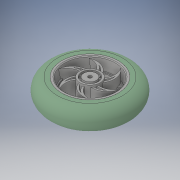
# Autodesk Inventor part: Wheel Hub
Saved by Autodesk Inventor 2018 (Build 220112000, 112)
## iProperties
Created: 2018-03-28
Part Number: Wheel Hub
Material: Generic
Document SubType Name: Modeling
Designer: Ajith Thomas
Density: 1 g/cm^3
Appearance: Default
Author: Ajith Thomas
Autodesk Inventor part; units mm, degrees
ref_plane "YZ Plane" through (0, 0, 0) normal (1, 0, 0) x (0, 1, 0)
sketch "Sketch1" plane through (0, 0, 0) normal (0, 1, 0) x (-1, 0, 0)
  circle A0 centre (0, 0) radius 23.5
  dimension "d0" = 47
  constraints: 1 centre point, 1 coincident
  measures "d0" diameter of A0
extrude "Extrusion1" add sketch "Sketch1" along normal blind 19
sketch "Sketch2" plane through (0, 19, 0) normal (0, 1, 0) x (1, 0, 0)
  circle A0 centre (0, 0) radius 21.25
  dimension "d3" = 42.5
  constraints: 1 centre point, 1 coincident
  measures "d3" diameter of A0
extrude "Extrusion2" cut sketch "Sketch2" against normal blind 19
sketch "Sketch3" plane through (0, 19, 0) normal (0, 1, 0) x (1, 0, 0)
  circle A0 centre (0, 0) radius 5.25
  dimension "d6" = 10.5
  constraints: 1 centre point, 1 coincident
  measures "d6" diameter of A0
extrude "Extrusion3" add sketch "Sketch3" against normal blind 19
sketch "Sketch4" plane through (0, 19, 0) normal (0, 1, 0) x (1, 0, 0)
  circle A0 centre (0, 0) radius 1.5
  dimension "d9" = 3
  constraints: 1 centre point, 1 coincident
  measures "d9" diameter of A0
extrude "Extrusion4" cut sketch "Sketch4" against normal blind 19
ref_plane "Work Plane1" through (0, 9.5, 0) normal (0, 1, 0) x (1, 0, 0)
sketch "Sketch5" plane through (0, 9.5, 0) normal (0, 1, 0) x (1, 0, 0)
  circle A0 centre (0, 0) radius 5.25 projected
  circle A1 centre (0, 0) radius 21.25 projected
  line L0 (-21.25, 0) -> (0, 0) construction
  line L1 (0, 0) -> (21.25, 0) construction
  circle A2 centre (0, 0) radius 1.5 construction
  line L2 (0, -21.25) -> (0, 0) construction
  line L3 (0, 0) -> (0, 21.25) construction
  arc A3 (-2.2887, 4.7249) -> (-15.5928, 14.437) centre (-13.6129, 3.1808) ccw
  arc A4 (2.8284, 4.4229) -> (-15.5928, 14.437) centre (-10.0016, 2.772) ccw
  arc A5 (2.8284, 4.4229) -> (-2.2887, 4.7249) centre (0, 0) ccw
  arc A6 (-2.4162, 4.661) -> (-5.2362, 0.3804) centre (0, 0) ccw
  arc A7 (-5.2362, 0.3804) -> (-20.2992, -6.2853) centre (-9.5611, -10.1987) ccw
  arc A8 (-2.4162, 4.661) -> (-20.2992, -6.2853) centre (-7.4014, -7.2756) ccw
  arc A9 (-5.2446, 0.238) -> (-2.9475, -4.3445) centre (0, 0) ccw
  arc A10 (-2.9475, -4.3445) -> (-4.7064, -20.7223) centre (4.0518, -13.3795) ccw
  arc A11 (-5.2446, 0.238) -> (-4.7064, -20.7223) centre (2.6002, -10.0476) ccw
  arc A12 (-2.8284, -4.4229) -> (2.2887, -4.7249) centre (0, 0) ccw
  arc A13 (2.2887, -4.7249) -> (15.5928, -14.437) centre (13.6129, -3.1808) ccw
  arc A14 (-2.8284, -4.4229) -> (15.5928, -14.437) centre (10.0016, -2.772) ccw
  arc A15 (2.4162, -4.661) -> (5.2362, -0.3804) centre (0, 0) ccw
  arc A16 (5.2362, -0.3804) -> (20.2992, 6.2853) centre (9.5611, 10.1987) ccw
  arc A17 (2.4162, -4.661) -> (20.2992, 6.2853) centre (7.4014, 7.2756) ccw
  arc A18 (5.2446, -0.238) -> (2.9475, 4.3445) centre (0, 0) ccw
  arc A19 (2.9475, 4.3445) -> (4.7064, 20.7223) centre (-4.0518, 13.3795) ccw
  arc A20 (5.2446, -0.238) -> (4.7064, 20.7223) centre (-2.6002, 10.0476) ccw
  dimension "d14" = 360
  constraints: 43 point on circle, 18 centre point, 8 end point, 2 point on line, 1 horizontal, 1 vertical, 55 other
extrude "Extrusion5" add sketch "Sketch5" along normal mid plane 16 contours A0 A19 A20 | A0 A3 A4 | A16 A17 A0 | A0 A7 A8 | A13 A14 A0 | A11 A0 A10
sketch "Sketch6" plane through (0, 17.5, 0) normal (0, 1, 0) x (1, 0, 0)
  arc A0 (-2.2887, 4.7249) -> (-15.5928, 14.437) centre (-13.6129, 3.1808) ccw projected
  arc A1 (2.8284, 4.4229) -> (-15.5928, 14.437) centre (-10.0016, 2.772) ccw projected
  arc A2 (2.8284, 4.4229) -> (-2.2887, 4.7249) centre (0, 0) ccw projected
  arc A3 (2.8284, 4.4229) -> (-15.5928, 14.437) centre (-10.0016, 2.772) ccw projected
  arc A4 (-2.2887, 4.7249) -> (-15.5928, 14.437) centre (-13.6129, 3.1808) ccw projected
  arc A5 (-0.9458, 5.1641) -> (-6.2823, 13.6998) centre (-13.6129, 3.1808) ccw
  arc A6 (1.3079, 5.0845) -> (-6.2823, 13.6998) centre (-10.0016, 2.772) ccw
  arc A7 (1.3079, 5.0845) -> (-0.9458, 5.1641) centre (0, 0) ccw
  arc A8 (-3.7494, 3.6749) -> (-4.9452, 1.7629) centre (0, 0) ccw
  arc A9 (-4.9452, 1.7629) -> (-15.0055, 1.4093) centre (-9.5611, -10.1987) ccw
  arc A10 (-3.7494, 3.6749) -> (-15.0055, 1.4093) centre (-7.4014, -7.2756) ccw
  arc A11 (-5.0572, -1.4096) -> (-3.9993, -3.4012) centre (0, 0) ccw
  arc A12 (-3.9993, -3.4012) -> (-8.7232, -12.2905) centre (4.0518, -13.3795) ccw
  arc A13 (-5.0572, -1.4096) -> (-8.7232, -12.2905) centre (2.6002, -10.0476) ccw
  arc A14 (-1.3079, -5.0845) -> (0.9458, -5.1641) centre (0, 0) ccw
  arc A15 (0.9458, -5.1641) -> (6.2823, -13.6998) centre (13.6129, -3.1808) ccw
  arc A16 (-1.3079, -5.0845) -> (6.2823, -13.6998) centre (10.0016, -2.772) ccw
  arc A17 (3.7494, -3.6749) -> (4.9452, -1.7629) centre (0, 0) ccw
  arc A18 (4.9452, -1.7629) -> (15.0055, -1.4093) centre (9.5611, 10.1987) ccw
  arc A19 (3.7494, -3.6749) -> (15.0055, -1.4093) centre (7.4014, 7.2756) ccw
  arc A20 (5.0572, 1.4096) -> (3.9993, 3.4012) centre (0, 0) ccw
  arc A21 (3.9993, 3.4012) -> (8.7232, 12.2905) centre (-4.0518, 13.3795) ccw
  arc A22 (5.0572, 1.4096) -> (8.7232, 12.2905) centre (-2.6002, 10.0476) ccw
  dimension "d20" = 360
  constraints: 38 point on circle, 18 centre point, 55 other
extrude "Extrusion6" cut sketch "Sketch6" against normal blind 5.5 contours A5 A6 A2 | A8 A9 A10 | A11 A12 A13 | A14 A15 A16 | A17 A18 A19 | A20 A21 A22
ref_plane "Work Plane2" through (0, 9.5, 0) normal (0, 1, 0) x (1, 0, 0)
mirror "Mirror1" about plane through (0, 9.5, 0) normal (0, 1, 0) of "Extrusion6"
sketch "Sketch7" plane through (0, 0, 0) normal (0, 0, 1) x (1, 0, 0)
  line L0 (-21.25, 19) -> (-21.25, 0) projected
  line L1 (-21.25, 9.5) -> (-19.25, 9.5) construction
  line L2 (-19.25, 9.5) -> (-19.25, 10)
  line L3 (-19.25, 9.5) -> (-19.25, 9)
  line L4 (-19.25, 10) -> (-20.25, 10)
  line L5 (-19.25, 9) -> (-20.25, 9)
  line L6 (-20.25, 10) -> (-21.25, 19)
  line L7 (21.25, 0) -> (-21.25, 0) projected
  line L8 (-20.25, 9) -> (-21.25, 0)
  line L9 (-21.25, 19) -> (-21.25, 0)
  line L10 (-5.25, 19) -> (5.25, 19) projected
  line L11 (0, 19) -> (0, 0) construction
  line L12 (-5.25, 0) -> (5.25, 0) projected
  dimension "d24" = 2
  dimension "d25" = 0.5
  dimension "d26" = 0.5
  dimension "d27" = 1
  dimension "d28" = 1
  constraints: 18 end point, 3 horizontal, 2 midpoint, 2 vertical, 1 collinear, 1 perpendicular
  measures "d24" distance of L1.start L1.end
  measures "d25" distance of L1.end L2.end
  measures "d26" distance of L1.end L3.end
  measures "d27" distance of L2.end L4.end
  measures "d28" distance of L3.end L5.end
revolve "Revolution1" add sketch "Sketch7" angle 360 about axis through (0, 19, 0) along (0, -1, 0)
sketch "Sketch8" plane through (0, 19, 0) normal (0, 1, 0) x (1, 0, 0)
  circle A0 centre (0, 0) radius 8.5
  circle A1 centre (0, 0) radius 7
  dimension "d30" = 17
  dimension "d31" = 14
  constraints: 2 centre point, 2 coincident
  measures "d30" diameter of A0
  measures "d31" diameter of A1
extrude "Extrusion7" add sketch "Sketch8" against normal blind 19
sketch "Sketch9" plane through (0, 10, 0) normal (0, 1, 0) x (0.7381754, 0, -0.6746088)
  arc A0 (-7.7766, 3.4314) -> (-17.5475, -11.6872) centre (-4.8588, -9.171) ccw projected
  arc A1 (-16.3983, 10.0826) -> (-17.696, -7.5771) centre (0, 0) ccw projected
  arc A2 (-19.1982, -1.4108) -> (-15.7232, -2.1496) centre (-17.2118, -0.6095) ccw
  arc A3 (-15.7232, -2.1496) -> (-17.696, -7.5771) centre (-4.8588, -9.171) ccw
  arc A4 (-19.1982, -1.4108) -> (-17.696, -7.5771) centre (0, 0) ccw
  arc A5 (-8.3773, -17.3316) -> (-6, -14.6914) centre (-8.0781, -15.2106) ccw
  arc A6 (-8.3773, -17.3316) -> (-2.286, -19.1138) centre (0, 0) ccw
  arc A7 (-6, -14.6914) -> (-2.286, -19.1138) centre (5.5129, -8.7933) ccw
  arc A8 (10.8209, -15.9208) -> (9.7232, -12.5419) centre (9.1337, -14.6011) ccw
  arc A9 (10.8209, -15.9208) -> (15.41, -11.5366) centre (0, 0) ccw
  arc A10 (9.7232, -12.5419) -> (15.41, -11.5366) centre (10.3717, 0.3777) ccw
  arc A11 (19.1982, 1.4108) -> (15.7232, 2.1496) centre (17.2118, 0.6095) ccw
  arc A12 (19.1982, 1.4108) -> (17.696, 7.5771) centre (0, 0) ccw
  arc A13 (15.7232, 2.1496) -> (17.696, 7.5771) centre (4.8588, 9.171) ccw
  arc A14 (8.3773, 17.3316) -> (6, 14.6914) centre (8.0781, 15.2106) ccw
  arc A15 (8.3773, 17.3316) -> (2.286, 19.1138) centre (0, 0) ccw
  arc A16 (6, 14.6914) -> (2.286, 19.1138) centre (-5.5129, 8.7933) ccw
  arc A17 (-10.8209, 15.9208) -> (-9.7232, 12.5419) centre (-9.1337, 14.6011) ccw
  arc A18 (-10.8209, 15.9208) -> (-15.41, 11.5366) centre (0, 0) ccw
  arc A19 (-9.7232, 12.5419) -> (-15.41, 11.5366) centre (-10.3717, -0.3777) ccw
  dimension "d36" = 360
  constraints: 38 point on circle, 18 centre point, 2 concentric, 55 other
extrude "Extrusion8" add sketch "Sketch9" against normal blind 1
sketch "Sketch10" plane through (0, 9.5, 0) normal (0, 1, 0) x (1, 0, 0)
  circle A0 centre (0, 0) radius 7.4396
  constraints: 1 centre point, 1 coincident
extrude "Extrusion9" add sketch "Sketch10" along normal mid plane 1
sketch "Sketch11" plane through (0, 0, 0) normal (0, 0, 1) x (1, 0, 0)
  line L0 (-5.25, 19) -> (5.25, 19) construction
  line L1 (0, 19) -> (0, 0) construction
  line L2 (0.7557, 7) -> (0.7557, 1.5) construction
  line L3 (23.5, 0) -> (23.5, 19) construction
  line L4 (23.5, 9.5) -> (35, 9.5) construction
  line L5 (-23.5, 0) -> (23.5, 0) projected
  line L6 (23.5, 19) -> (-23.5, 19) projected
  arc A0 (27.1522, 0) -> (27.1522, 19) centre (25.3261, 9.5) ccw
  line L7 (23.5, 0) -> (27.1522, 0)
  line L8 (23.5, 19) -> (27.1522, 19)
  line L9 (23.5, 19) -> (23.5, 0)
  dimension "d42" = 35
  constraints: 10 end point, 3 point on circle, 2 horizontal, 2 midpoint, 2 perpendicular, 1 centre point, 1 parallel
  measures "d42" distance from line of L1 L4.end
revolve "Revolution2" add sketch "Sketch11" angle 360 about axis through (0, 19, 0) along (0, -1, 0) separate body
chamfer "Chamfer1" distance 0.6 angle 45 2 edges at (21.25, 19, 0) (21.25, 0, 0)
body "Solid1"
body "Solid2"
